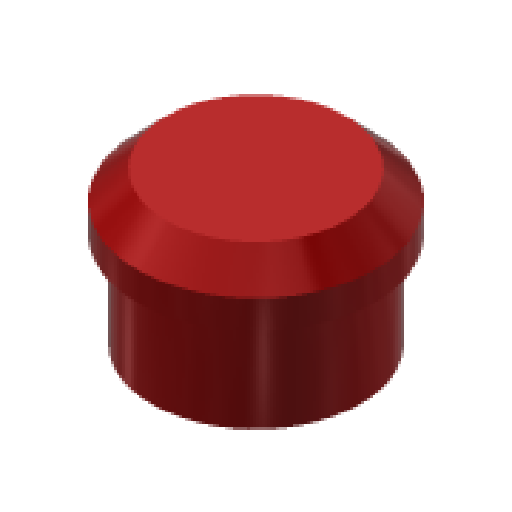
# Autodesk Inventor part: E-Stop Dummy
Saved by Autodesk Inventor 2023.2 (Build 272271000, 271)
## iProperties
Created: 2023-02-07
Part Number: E-Stop Dummy
Material: ABS Plastic
Document SubType Name: Modeling
Designer: remop
Density: 1.06 g/cm^3
Appearance: Smooth - Red
Author: remop
Autodesk Inventor part; units mm, degrees
ref_plane "YZ Plane" through (0, 0, 0) normal (1, 0, 0) x (0, 1, 0)
ref_plane "XZ Plane" through (0, 0, 0) normal (0, 1, 0) x (-1, 0, 0)
ref_plane "XY Plane" through (0, 0, 0) normal (0, 0, 1) x (1, 0, 0)
sketch "Sketch1" plane through (0, 0, 0) normal (0, 0, 1) x (1, 0, 0)
  line L0 (0, 0) -> (0, 23.6158)
  line L1 (0, 0) -> (11, 0)
  line L2 (11, 0) -> (11, 10)
  line L3 (11, 10) -> (15, 10)
  line L4 (15, 10) -> (15, 13)
  line L5 (15, 13) -> (10, 18)
  line L6 (10, 18) -> (0, 18)
  dimension "d0" = 45
  dimension "d1" = 22
  dimension "d2" = 30
  dimension "d3" = 10
  dimension "d4" = 3
  dimension "d5" = 5
  constraints: 14 end point, 4 perpendicular, 1 horizontal, 1 point on line, 1 vertical
  measures "d0" angle of L6 L5
  measures "d1" diameter of L2 L0
  measures "d2" diameter of L4 L0
  measures "d3" distance of L1.end L2.end
  measures "d4" distance of L3.end L4.end
  measures "d5" horizontal distance of L4.end L5.end
revolve "Revolution1" add sketch "Sketch1" angle 360 about axis through (0, 0, 0) along (0, 1, 0)
body "Solid1"
